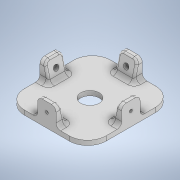
# Autodesk Inventor part: 鋁擠加強肋(上層)
Saved by Autodesk Inventor 2021 (Build 250183000, 183)
## iProperties
Created: 2023-02-15
Part Number: 鋁擠加強肋(上層)
Material: 一般
Document SubType Name: Modeling
Designer: brian
Density: 1 g/cm^3
Appearance: 預設
Author: brian
Autodesk Inventor part; units mm, degrees
ref_plane "YZ Plane" through (0, 0, 0) normal (1, 0, 0) x (0, 1, 0)
sketch "草圖1" plane through (0, 0, 0) normal (0, 1, 0) x (-1, 0, 0)
  line L0 (-44.5, 47) -> (44.5, 47)
  line L1 (44.5, 47) -> (44.5, -47)
  line L2 (44.5, -47) -> (-44.5, -47)
  line L3 (-44.5, -47) -> (-44.5, 47)
  line L4 (-44.5, 47) -> (44.5, -47) construction
  line L5 (44.5, 47) -> (-44.5, -47) construction
  point P0 (0, 0)
  dimension "d0" = 89
  dimension "d1" = 94
  constraints: 12 end point, 2 midpoint, 2 parallel, 1 horizontal, 1 perpendicular
  measures "d0" distance of L1.end L2.end
  measures "d1" distance of L0.end L1.end
extrude "擠出1" add sketch "草圖1" along normal blind 5
sketch "草圖2" plane through (0, 5, 0) normal (0, 1, 0) x (1, 0, 0)
  circle A0 centre (0, 0) radius 10
  dimension "d4" = 20
  constraints: 1 centre point, 1 coincident
  measures "d4" diameter of A0
extrude "擠出2" cut sketch "草圖2" against normal through all
sketch "草圖3" plane through (0, 0, 0) normal (1, 0, 0) x (0, 1, 0)
  line L0 (5, 47) -> (5, -47) projected
  line L1 (5, 47) -> (25, 47)
  line L2 (25, 47) -> (25, 42)
  line L3 (25, 42) -> (5, 37)
  point P0 (0, 0)
  dimension "d7" = 20
  dimension "d8" = 5
  dimension "d9" = 10
  constraints: 6 end point, 1 horizontal, 1 perpendicular, 1 point on line
  measures "d7" distance of L0.start L1.end
  measures "d8" distance of L1.end L2.end
  measures "d9" distance of L0.start L3.end
extrude "擠出3" add sketch "草圖3" along normal mid plane 20
ref_plane "工作平面1" through (0, 5, 37) normal (0, 0, 1) x (1, 0, 0)
sketch "草圖4" plane through (0, 5, 37) normal (0, 0, 1) x (1, 0, 0)
  line L0 (-10, 20) -> (10, 20) projected
  line L1 (-10, 20) -> (-10, 0) projected
  point P0 (0, -5)
  point P1 (0, 10)
  point P2 (0, 20)
  point P3 (-10, 10)
  constraints: 2 midpoint, 1 horizontal alignment, 1 vertical alignment
hole "孔1" at (0, 15, 37) direction (0, 0, 1) diameter 3.2 end through all counterbore diameter 5.8 counterbore depth 5
mirror "鏡射1" about plane through (0, 0, 0) normal (0, 0, 1) of "孔1", "擠出3"
sketch "草圖5" plane through (0, 0, 0) normal (0, 0, 1) x (1, 0, 0)
  line L0 (-44.5, 0) -> (-44.5, 5) projected
  line L1 (-44.5, 5) -> (-44.5, 25)
  line L2 (-44.5, 25) -> (-39.5, 25)
  line L3 (-39.5, 25) -> (-34.5, 5)
  line L4 (-44.5, 5) -> (-10, 5) projected
  point P0 (0, 0)
  dimension "d19" = 20
  dimension "d20" = 5
  dimension "d21" = 10
  constraints: 6 end point, 1 perpendicular, 1 point on line, 1 vertical
  measures "d19" distance of L0.end L1.end
  measures "d20" distance of L1.end L2.end
  measures "d21" distance of L0.end L3.end
extrude "擠出4" add sketch "草圖5" along normal mid plane 20
ref_plane "工作平面2" through (-34.5, 5, 0) normal (-1, 0, 0) x (0, 0, 1)
sketch "草圖6" plane through (-34.5, 5, 0) normal (-1, 0, 0) x (0, 0, 1)
  line L0 (-10, 20) -> (10, 20) projected
  line L1 (-10, 20) -> (-10, 0) projected
  point P0 (0, -5)
  point P1 (0, 10)
  point P2 (0, 20)
  point P3 (-10, 10)
  constraints: 2 midpoint, 1 horizontal alignment, 1 vertical alignment
hole "孔2" at (-34.5, 15, 0) direction (-1, 0, 0) diameter 3.2 end through all counterbore diameter 5.8 counterbore depth 5
mirror "鏡射2" about plane through (0, 0, 0) normal (1, 0, 0) of "擠出4", "孔2"
fillet "圓角1" radius 20 4 edges at (44.5, 2.5, -47) (44.5, 2.5, 47) (-44.5, 2.5, -47) (-44.5, 2.5, 47)
fillet "圓角2" radius 5 20 edges at (10, 5, 42) (39.5, 5, 10) (39.5, 5, -10) (10, 5, -42) (-10, 5, -42) (-39.5, 5, -10) (-39.5, 5, 10) (-10, 5, 42) (-34.5, 5, 0) (0, 5, 37) (34.5, 5, 0) (0, 5, -37) (-10, 25, -44.5) (10, 25, -44.5) (42, 25, -10) (42, 25, 10) (10, 25, 44.5) (-10, 25, 44.5) (-42, 25, -10) (-42, 25, 10)
fillet "圓角2" radius 2 12 edges at (10, 15, 39.5) (-10, 15, 39.5) (0, 25, 42) (-37, 15, 10) (-39.5, 25, 0) (-37, 15, -10) (10, 15, -39.5) (0, 25, -42) (-10, 15, -39.5) (37, 15, 10) (39.5, 25, 0) (37, 15, -10)
